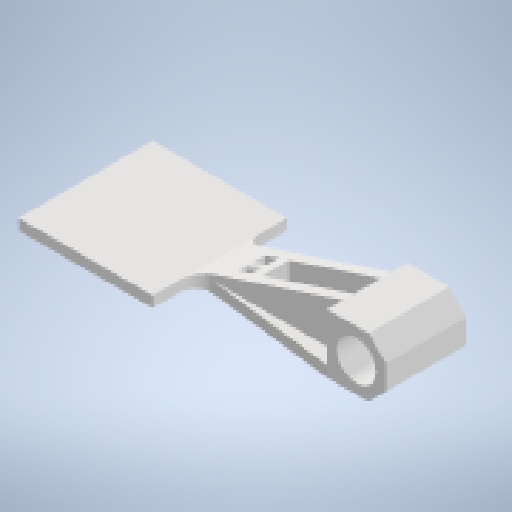
# Autodesk Inventor part: Brazo catapulta
Saved by Autodesk Inventor 2024 (Build 280153000, 153)
## iProperties
Created: 2025-03-01
Part Number: Brazo catapulta
Material: Genérico
Document SubType Name: Modeling
Designer: sergi
Density: 1 g/cm^3
Appearance: Valor por defecto
Author: sergi
Autodesk Inventor part; units mm, degrees
ref_plane "YZ Plane" through (0, 0, 0) normal (1, 0, 0) x (0, 1, 0)
ref_plane "XZ Plane" through (0, 0, 0) normal (0, 1, 0) x (-1, 0, 0)
ref_plane "XY Plane" through (0, 0, 0) normal (0, 0, 1) x (1, 0, 0)
sketch "Boceto1" plane through (0, 0, 0) normal (0, 1, 0) x (-1, 0, 0)
  line L0 (0, 0) -> (22, 0)
  line L1 (22, 0) -> (22, 30)
  line L2 (22, 30) -> (0, 30)
  line L3 (0, 30) -> (0, 0)
  dimension "d0" = 22
  dimension "d1" = 30
  constraints: 8 end point, 2 parallel, 1 horizontal, 1 perpendicular
  measures "d0" distance of L2.end L1.end
  measures "d1" distance of L1.end L0.end
extrude "Extrusión1" add sketch "Boceto1" along normal blind 22
sketch "Boceto2" plane through (-22, 0, 30) normal (0, 0, 1) x (1, 0, 0)
  line L0 (0, 0) -> (22, 0) projected
  line L1 (22, 0) -> (22, 22) projected
  line L2 (0, 22) -> (22, 22) projected
  line L3 (0, 0) -> (0, 22) projected
  line L4 (22, 22) -> (0, 0)
  circle A0 centre (11, 11) radius 7.3
  dimension "d35" = 50
  dimension "d4" = 14.6
  constraints: 2 end point, 1 centre point, 1 midpoint
  measures "d4" diameter of A0
extrude "Extrusión2" cut sketch "Boceto2" against normal through all contours A0 L4 | L4 A0
chamfer "Chaflán1" distance 6.5 angle 45 2 edges at (0, 22, 15) (0, 0, 15)
sketch "Boceto3" plane through (-22, 0, 30) normal (0, 0, 1) x (1, 0, 0)
  line L0 (-84.9, -39.92) -> (20.1, -39.92) projected
  line L1 (20.1, -39.92) -> (20.1, -9.92) projected
  line L2 (-84.9, -9.92) -> (20.1, -9.92) projected
  line L3 (-84.9, -39.92) -> (-84.9, -9.92) projected
  line L4 (-88.7564, 6.9) -> (-92.3631, 6.9) projected
  line L5 (22, 6.5) -> (15.5, 0) projected
  line L6 (22, 6.5) -> (22, 15.5) projected
  line L7 (15.5, 22) -> (22, 15.5) projected
  line L8 (0, 22) -> (15.5, 22) projected
  line L9 (0, 0) -> (0, 22) projected
  line L10 (0, 0) -> (15.5, 0) projected
  circle A0 centre (11, 11) radius 7.3 projected
  line L11 (0, 0) -> (-84.9, 0)
  line L12 (0, 0) -> (-104.9, 0)
  line L13 (-104.9, 0) -> (-104.9, 4)
  line L14 (-104.9, 4) -> (0, 4)
  line L15 (0, 4) -> (0, 0)
  line L16 (-104.9, 4) -> (-54.9, 4)
  line L17 (-104.9, 4) -> (-54.9, 4) construction
  line L18 (-54.9, 4) -> (0, 22)
  point P0 (22, 0)
  point P1 (-54.9, 4)
  point P2 (0, 4)
  point P3 (0, 4)
  dimension "d33" = 104.9
  dimension "d34" = 4
  dimension "d35" = 50
  constraints: 16 end point, 3 horizontal, 2 collinear, 2 parallel, 1 perpendicular
  measures "d33" distance of L13.end L14.end
  measures "d34" distance of L12.end L13.end
  measures "d35" distance of L13.end L16.end
extrude "Extrusión3" add sketch "Boceto3" against normal up to surface (30 mm away) contours L11 L12 L13 L14 L9 | L14 L18 L9
sketch "Boceto6" plane through (0, 6.5, 30) normal (0, 0, 1) x (1, 0, 0)
  line L0 (0, 0) -> (-6.5, -6.5) projected
  line L1 (0, 0) -> (0, 9) projected
  line L2 (-6.5, 15.5) -> (0, 9) projected
  line L3 (-22, 15.5) -> (-6.5, 15.5) projected
  circle A0 centre (-11, 4.5) radius 7.3 projected
  line L4 (-106.9, -2.5) -> (-76.9, -2.5)
  line L5 (-76.9, -2.5) -> (-76.9, -6.5)
  line L6 (-22, 15.5) -> (-22, -6.5)
  line L7 (-126.9, -6.5) -> (-6.5, -6.5) projected
  line L8 (-22, 15.5) -> (-76.9, -2.5) projected
  line L9 (-76.9, -2.5) -> (-126.9, -2.5) projected
  line L10 (-126.9, -2.5) -> (-126.9, -6.5) projected
  point P0 (0, -6.5)
  dimension "d26" = 30
  constraints: 6 end point
  measures "d26" distance of L4.start L4.end
extrude "Extrusión6" cut sketch "Boceto6" against normal blind 6 contours L7 L5 L8 L6
sketch "Boceto7" plane through (0, 6.5, 0) normal (0, 0, -1) x (-1, 0, 0)
  line L0 (36.9, -16.42) -> (1.9, -16.42) projected
  line L1 (76.9, -6.5) -> (76.9, -2.5) projected
  line L2 (22, -6.5) -> (76.9, -6.5) projected
  line L3 (22, 15.5) -> (22, -6.5) projected
  line L4 (76.9, -2.5) -> (22, 15.5) projected
  point P0 (0, -6.5)
extrude "Extrusión7" cut sketch "Boceto7" against normal blind 6 from surface at 0
sketch "Boceto8" plane through (0, 0, 0) normal (0, -1, 0) x (1, 0, 0)
  line L0 (-60.1, 26) -> (-60.1, 4) projected
  line L1 (-66.1, 19.8661) -> (-66.1, 15.3661) projected
  line L2 (-66.1, 14.6339) -> (-66.1, 10.1339) projected
  line L3 (-65.1, 26.6) -> (-65.1, 3.4) projected
  line L4 (-65.1, 26.6) -> (-65.1, 3.4) projected
  line L5 (-22, 24) -> (-76.9, 24) projected
  line L6 (-22, 6) -> (-76.9, 6) projected
  line L7 (-22, 20) -> (-76.9, 20)
  line L8 (-22, 10) -> (-76.9, 10)
  line L9 (-65.1, 20) -> (-65.1, 17)
  line L10 (-65.1, 17) -> (-60.1, 17)
  line L11 (-65.1, 10) -> (-65.1, 13)
  line L12 (-65.1, 13) -> (-60.1, 13)
  point P0 (0, 0)
  point P1 (-60.1, 10)
  point P2 (-60.1, 20)
  dimension "d37" = 4
  dimension "d38" = 4
  dimension "d39" = 3
  dimension "d40" = 3
  constraints: 12 end point, 8 point on line, 2 parallel, 2 perpendicular
  measures "d37" distance between parallel lines of L5 L7
  measures "d38" distance between parallel lines of L6 L8
  measures "d39" distance of L9.start L9.end
  measures "d40" distance of L11.start L11.end
extrude "Extrusión8" cut sketch "Boceto8" against normal through all contours L10 L3 L7 L0 | L0 L8 L3 L12
fillet "Empalme2" radius 2 4 edges at (-62.6, 8.6885, 13) (-62.6, 8.6885, 17) (-62.6, 0, 20) (-62.6, 0, 10)
fillet "Empalme3" radius 6 2 edges at (-76.9, 2, 24) (-76.9, 2, 6)
sketch "Boceto9" plane through (0, 0, 0) normal (0, -1, 0) x (1, 0, 0)
  line L0 (-65.1, 8) -> (-65.1, 13) projected
  line L1 (-65.1, 13) -> (-60.1, 13) projected
  line L2 (-60.1, 13) -> (-60.1, 8) projected
  line L3 (-65.1, 8) -> (-60.1, 8) projected
  line L4 (-60.1, 22) -> (-60.1, 17) projected
  line L5 (-60.1, 17) -> (-65.1, 17) projected
  line L6 (-65.1, 17) -> (-65.1, 22) projected
  line L7 (-60.1, 22) -> (-65.1, 22) projected
  line L8 (-22, 6) -> (-22, 0) projected
  line L9 (-6.5, 0) -> (-22, 0) projected
  line L10 (-6.5, 30) -> (-6.5, 0) projected
  line L11 (-22, 30) -> (-6.5, 30) projected
  line L12 (-22, 30) -> (-22, 24) projected
  line L13 (-22, 24) -> (-70.9, 24) projected
  arc A0 (-76.9, 30) -> (-70.9, 24) centre (-70.9, 30) ccw projected
  line L14 (-126.9, 30) -> (-76.9, 30) projected
  line L15 (-76.9, 0) -> (-126.9, 0) projected
  arc A1 (-70.9, 6) -> (-76.9, 0) centre (-70.9, 0) ccw projected
  line L16 (-22, 6) -> (-70.9, 6) projected
  line L17 (-70.9, 20) -> (-18, 20)
  line L18 (-18, 20) -> (-18, 26)
  line L19 (-18, 26) -> (-10.5, 26)
  line L20 (-10.5, 26) -> (-10.5, 4)
  line L21 (-10.5, 4) -> (-18, 4)
  line L22 (-18, 4) -> (-18, 10)
  line L23 (-18, 10) -> (-70.9, 10)
  arc A2 (-70.9, 10) -> (-80.0652, 4) centre (-70.9, 0) ccw
  line L24 (-80.0652, 4) -> (-102.9, 4)
  line L25 (-102.9, 4) -> (-102.9, 26)
  line L26 (-102.9, 26) -> (-80.0652, 26)
  arc A3 (-80.0652, 26) -> (-70.9, 20) centre (-70.9, 30) ccw
  line L27 (-56.1, 13) -> (-56.1, 26)
  line L28 (-56.1, 26) -> (-69.1, 26)
  line L29 (-69.1, 26) -> (-69.1, 13)
  line L30 (-69.1, 13) -> (-56.1, 13)
  line L31 (-56.1, 4) -> (-56.1, 17)
  line L32 (-56.1, 17) -> (-69.1, 17)
  line L33 (-69.1, 17) -> (-69.1, 4)
  line L34 (-69.1, 4) -> (-56.1, 4)
  line L35 (-22, 24) -> (-22, 6)
  line L36 (-22, 15) -> (-56.1, 17)
  line L37 (-126.9, 30) -> (-126.9, 0) projected
  point P0 (0, 0)
  point P1 (-22, 20)
  point P2 (-56.1, 20)
  point P3 (-56.1, 10)
  point P4 (-22, 10)
  dimension "d45" = 4
  dimension "d46" = 4
  constraints: 40 end point, 4 point on circle, 2 centre point, 1 midpoint, 1 vertical, 15 other
  measures "d45" distance between parallel lines of L4 L27
  measures "d46" distance between parallel lines of L2 L31
extrude "Extrusión9" cut sketch "Boceto9" against normal through all contours L31 L27 L36 L35 L23 | L27 L17 L35 L36
sketch "Boceto10" plane through (0, 0, 0) normal (0, -1, 0) x (1, 0, 0)
  line L0 (-56.1, 10) -> (-56.1, 20) projected
  line L1 (-56.1, 20) -> (-22, 20) projected
  line L2 (-22, 20) -> (-22, 10) projected
  line L3 (-22, 10) -> (-56.1, 10) projected
  line L4 (-65.1, 8) -> (-65.1, 13) projected
  line L5 (-65.1, 13) -> (-60.1, 13) projected
  line L6 (-60.1, 13) -> (-60.1, 8) projected
  line L7 (-65.1, 8) -> (-60.1, 8) projected
  line L8 (-60.1, 22) -> (-60.1, 17) projected
  line L9 (-60.1, 17) -> (-65.1, 17) projected
  line L10 (-65.1, 17) -> (-65.1, 22) projected
  line L11 (-60.1, 22) -> (-65.1, 22) projected
  line L12 (-22, 6) -> (-22, 0) projected
  line L13 (-6.5, 0) -> (-22, 0) projected
  line L14 (-6.5, 30) -> (-6.5, 0) projected
  line L15 (-22, 30) -> (-6.5, 30) projected
  line L16 (-22, 30) -> (-22, 24) projected
  line L17 (-22, 24) -> (-70.9, 24) projected
  arc A0 (-76.9, 30) -> (-70.9, 24) centre (-70.9, 30) ccw projected
  line L18 (-126.9, 30) -> (-76.9, 30) projected
  line L19 (-76.9, 0) -> (-126.9, 0) projected
  arc A1 (-70.9, 6) -> (-76.9, 0) centre (-70.9, 0) ccw projected
  line L20 (-22, 6) -> (-70.9, 6) projected
  line L21 (-22, 30) -> (-70.9, 24)
  line L22 (-22, 0) -> (-70.9, 6)
  line L23 (-126.9, 30) -> (-126.9, 0) projected
  point P0 (0, 0)
  constraints: 4 end point, 1 point on line
extrude "Extrusión10" add sketch "Boceto10" against normal blind 4 contours L12 L22 L20 | L16 L17 L21
sketch "Boceto11" plane through (-126.9, 0, 30) normal (0, 0, 1) x (1, 0, 0)
  line L0 (50, 0) -> (50, 4) projected
  line L1 (50, 4) -> (0, 4) projected
  line L2 (0, 4) -> (0, 0) projected
  line L3 (0, 0) -> (50, 0) projected
  point P0 (126.9, 0)
extrude "Extrusión11" add sketch "Boceto11" along normal blind 10
sketch "Boceto12" plane through (-126.9, 0, 0) normal (0, 0, -1) x (-1, 0, 0)
  line L0 (-50, 4) -> (-50, 0) projected
  line L1 (-50, 0) -> (0, 0) projected
  line L2 (0, 4) -> (0, 0) projected
  line L3 (-50, 4) -> (0, 4) projected
  point P0 (-126.9, 0)
extrude "Extrusión12" add sketch "Boceto12" along normal blind 10
sketch "Boceto13" plane through (-126.9, 4, 40) normal (0, 1, 0) x (1, 0, 0)
  line L0 (14.8369, 42.1331) -> (18.4436, 26.384) projected
  arc A0 (14.8369, 42.1331) -> (9.9631, 42.1331) centre (12.4, 41.575) ccw projected
  line L1 (6.3564, 26.384) -> (9.9631, 42.1331) projected
  arc A1 (6.3564, 26.384) -> (6.3564, 23.616) centre (12.4, 25) ccw projected
  line L2 (9.9631, 7.8669) -> (6.3564, 23.616) projected
  arc A2 (9.9631, 7.8669) -> (14.8369, 7.8669) centre (12.4, 8.425) ccw projected
  line L3 (18.4436, 23.616) -> (14.8369, 7.8669) projected
  arc A3 (18.4436, 23.616) -> (18.4436, 26.384) centre (12.4, 25) ccw projected
  circle A4 centre (12.4, 25) radius 1.55 projected
  line L4 (18.6, 44.075) -> (6.2, 44.075)
  line L5 (6.2, 44.075) -> (6.2, 5.925)
  line L6 (6.2, 5.925) -> (18.6, 5.925)
  line L7 (18.6, 5.925) -> (18.6, 44.075)
  line L8 (18.6, 44.075) -> (6.2, 5.925) construction
  line L9 (6.2, 44.075) -> (18.6, 5.925) construction
  line L10 (20, 45.075) -> (0, 45.075)
  line L11 (5.2, 45.075) -> (5.2, 4.925)
  line L12 (0, 4.925) -> (20, 4.925)
  line L13 (19.6, 4.925) -> (19.6, 45.075)
  line L14 (0, 50) -> (0, 0) projected
  line L15 (50, 0) -> (0, 0) projected
  line L16 (50, 10) -> (50, 0) projected
  line L17 (50, 10) -> (50, 40) projected
  line L18 (50, 40) -> (50, 50) projected
  line L19 (0, 50) -> (50, 50) projected
  line L20 (50, 0) -> (20, 0)
  line L21 (50, 0) -> (0, 0) projected
  line L22 (20, 0) -> (20, 50)
  point P0 (126.9, 40)
  dimension "d55" = 38.15
  dimension "d56" = 1
  dimension "d59" = 30
  constraints: 24 end point, 9 point on line, 4 parallel, 2 midpoint, 2 perpendicular, 1 horizontal
  measures "d55" distance of L5.end L4.end
  measures "d56" distance between parallel lines of L7 L13
  measures "d59" distance of L15.start L20.end
extrude "Extrusión13" cut sketch "Boceto13" against normal through all contours A0 L4 L7 A3 L0 | L0 A3 L3 A2 L2 A1 L1 A0 | A0 L1 A1 L5 L4 | L7 L6 A2 L3 A3 | A1 L2 A2 L6 L5 | A4 | L22 L12 L13 L10 | L13 L12 L11 L10 | L11 L12 L14 L10
